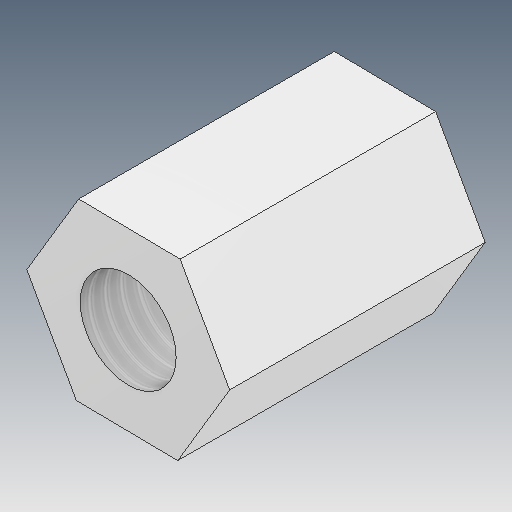
# Autodesk Inventor part: Espaciador para Electrónica 5mm
Saved by Autodesk Inventor 2020 (Build 240168000, 168)
## iProperties
Created: 2020-08-18
Part Number: Espaciador para Electrónica 5mm
Material: Acetal Resin, White
Document SubType Name: Modeling
Designer: Dante
Density: 1.425 g/cm^3
Appearance: Smooth - White
Author: Dante
Autodesk Inventor part; units mm, degrees
ref_plane "YZ Plane" through (0, 0, 0) normal (1, 0, 0) x (0, 1, 0)
ref_plane "XZ Plane" through (0, 0, 0) normal (0, 1, 0) x (-1, 0, 0)
ref_plane "XY Plane" through (0, 0, 0) normal (0, 0, 1) x (1, 0, 0)
sketch "Sketch1" plane through (0, 0, 0) normal (0, 0, 1) x (1, 0, 0)
  line L0 (-11.1101, 6.0966) -> (-9.5601, 3.3251)
  line L1 (-9.5601, 3.3251) -> (-11.1853, 0.5971)
  line L2 (-11.1853, 0.5971) -> (-14.3604, 0.6405)
  line L3 (-14.3604, 0.6405) -> (-15.9104, 3.412)
  line L4 (-15.9104, 3.412) -> (-14.2852, 6.14)
  line L5 (-14.2852, 6.14) -> (-11.1101, 6.0966)
  circle A0 centre (-12.7353, 3.3685) radius 1.5
  dimension "d0" = 5.5
  dimension "d1" = 3
  constraints: 12 end point, 1 centre point, 1 coincident, 13 other
  measures "d0" distance between parallel lines of L2 L5
  measures "d1" diameter of A0
extrude "Extrusion1" add sketch "Sketch1" along normal blind 8
thread "Thread2" size "M3x0.5" class "6H" standard "ANSI Metric M Profile" length 3.7
thread "Thread3" size "M3x0.5" class "6H" standard "ANSI Metric M Profile" length 3.7
body "Solid1"
